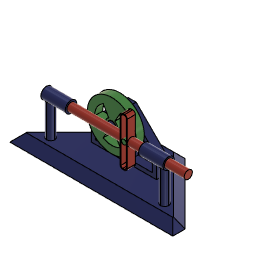
scotch yoke (Autodesk Fusion 360 design; units mm, degrees)
Autodesk Fusion 360 part; units mm, degrees
note: some values were not read from the file. Chosen so that the rebuilt part matches the saved one: which bodies a step acts on; which face or edge a step refers to; which pieces of a blend or face edit are solid. Set by a fixed rule: which sketch regions a step uses.
sketch "Base" plane through (0, 0, 0) normal (0, 0, 1) x (1, 0, 0) in component "Base"
  line L0 (10, -5) -> (-10, -5)
  line L1 (-10, -5) -> (-10, 5)
  line L2 (-10, 5) -> (10, 5)
  line L3 (10, 5) -> (10, -5)
  line L4 (10, -5) -> (-10, 5) construction
  line L5 (-10, -5) -> (10, 5) construction
  dimension "d9" = 20
  dimension "d10" = 10
  constraint horizontal L0
  constraint perpendicular L0 L1
  constraint parallel L0 L2
  constraint parallel L1 L3
  constraint coincident L4 origin
  constraint coincident L5 origin
  measures "d9" distance of L1.end L2.end
  measures "d10" distance of L0.end L1.end
extrude "Extrude1" add sketch "Base" along normal blind 1 makes body 1 in component "Base"
sketch "Crank holder" plane through (0, 0, 1) normal (0, 0, 1) x (-1, 0, 0) in component "Base"
  line L0 (-10, -5) -> (10, -5)
  line L1 (10, -5) -> (10, 5)
  line L2 (10, 5) -> (-10, 5)
  line L3 (-10, 5) -> (-10, -5)
  line L4 (0, 0) -> (4, 0)
  line L5 (4, 0) -> (4, -1)
  line L6 (4, -1) -> (0, -1)
  line L7 (0, -1) -> (0, 0)
  line L8 (-4, -1) -> (0, -1)
  line L9 (-4, 0) -> (-4, -1)
  line L10 (0, 0) -> (-4, 0)
  line L11 (-4, 0) -> (-4, 1.5) construction
  line L12 (-4, 1.5) -> (-4, 2.5) construction
  line L13 (-4, 2.5) -> (-7.5, 2.5) construction
  line L14 (-7.5, 2.5) -> (-7.5, 1.5) construction
  line L15 (-7.5, 1.5) -> (-4, 1.5) construction
  line L16 (4, 0) -> (4, 1.5) construction
  line L17 (4, 1.5) -> (4, 2.5) construction
  line L18 (4, 2.5) -> (7.5, 2.5) construction
  line L19 (7.5, 1.5) -> (4, 1.5) construction
  line L20 (7.5, 2.5) -> (7.5, 1.5) construction
  line L21 (-7.5, 1.5) -> (-6.5, 1.5)
  line L22 (-6.5, 1.5) -> (-6.5, 2.5)
  line L23 (-6.5, 2.5) -> (-7.5, 2.5)
  line L24 (-7.5, 2.5) -> (-7.5, 1.5)
  line L25 (7.5, 1.5) -> (6.5, 1.5)
  line L26 (6.5, 1.5) -> (6.5, 2.5)
  line L27 (6.5, 2.5) -> (7.5, 2.5)
  line L28 (7.5, 2.5) -> (7.5, 1.5)
  dimension "d15" = 4
  dimension "d16" = 1
  constraint horizontal L4
  constraint vertical L5
  constraint horizontal L6
  constraint vertical L7
  constraint coincident L4.start L7.end
  constraint symmetric L4.start L7 L10.start
  constraint symmetric L4.end L7 L9.start
  constraint symmetric L5.end L7 L8.start
  constraint symmetric L6.end L7 L8.end
  constraint perpendicular L10 L11
  constraint perpendicular L10 L12
  constraint perpendicular L12 L13
  constraint perpendicular L13 L14
  constraint perpendicular L12 L15
  constraint symmetric L7 L9.start L4.end
  constraint symmetric L7 L11.end L16.end
  constraint symmetric L7 L12.end L17.end
  constraint symmetric L7 L13.end L18.end
  constraint symmetric L7 L14.end L19.start
  constraint horizontal L21
  constraint vertical L22
  constraint horizontal L23
  constraint vertical L24
  constraint coincident L13 L22.end
  constraint horizontal L25
  constraint vertical L26
  constraint horizontal L27
  constraint vertical L28
  constraint coincident L18 L26.end
  measures "d15" distance of L4.start L4.end
  measures "d16" distance of L4.start L6.end
extrude "Extrude2" add sketch "Crank holder" along normal blind 6 contours L4 L5 L6 L7 | L7 L8 L9 L10 bodies 1 in component "Base"
chamfer "Chamfer1" distance 3.5 angle 45 2 edges at (4, 0.5, 7) (-4, 0.5, 7) on bodies 1 in component "Base"
sketch "Crank pin" plane through (0, 0, 0) normal (0, -1, 0) x (1, 0, 0) in component "Base"
  line L0 (-0.5, 7) -> (-4, 3.5)
  line L1 (-4, 3.5) -> (-4, 1)
  line L2 (-4, 1) -> (4, 1)
  line L3 (4, 1) -> (4, 3.5)
  line L4 (4, 3.5) -> (0.5, 7)
  line L5 (0.5, 7) -> (-0.5, 7)
  circle A0 centre (0, 5.5) radius 0.5
  line L6 (0, 5.5) -> (0, 1) construction
  dimension "d20" = 1
  constraint coincident A0.centre L6.start
  constraint midpoint L2 L6.end
  constraint perpendicular L2 L6
  measures "d20" diameter of A0
extrude "Extrude3" add sketch "Crank pin" along normal blind 1.5 contours A0 bodies 1 in component "Base"
extrude "Extrude4" add sketch "Crank holder" along normal blind 4.5 contours L21 L22 L23 L24 | L25 L26 L27 L28 bodies 1 in component "Base"
sketch "Crank" plane through (0, 0, 0) normal (0, -1, 0) x (1, 0, 0) in component "Crank"
  circle A0 centre (0, 5.5) radius 0.5
  line L0 (-0.5, 7) -> (-4, 3.5)
  line L1 (-4, 3.5) -> (-4, 1)
  line L2 (-4, 1) -> (4, 1)
  line L3 (4, 1) -> (4, 3.5)
  line L4 (4, 3.5) -> (0.5, 7)
  line L5 (0.5, 7) -> (-0.5, 7)
  circle A1 centre (0, 5.5) radius 3
  dimension "d25" = 6
  constraint concentric A0 A1
  measures "d25" diameter of A1
extrude "Extrude1'" add sketch "Crank" along normal blind 1.5 and the other way blind -0.5 separate body contours L0 L4 L5 A1 | L0 L4 L5 A1 makes body 2 in component "Crank"
sketch "holder" plane through (0, -0.5, 0) normal (0, 1, 0) x (-1, 0, 0) in component "Crank"
  circle A0 centre (0, 5.5) radius 0.5
  circle A1 centre (0, 5.5) radius 3
  circle A2 centre (0, 5.5) radius 0.5996
  dimension "d30" = 0.0996
extrude "Extrude2'" add sketch "holder" along normal blind 0.5 contours A2 bodies 2 in component "Crank"
move_face "OffsetFaces1" offset -0.02 1 faces at (0.4975, -1.1667, 5.4502) on bodies 2 in component "Crank"
sketch "pin" plane through (0, -1.5, 0) normal (0, -1, 0) x (1, 0, 0) in component "Crank"
  circle A0 centre (0, 5.5) radius 0.52
  circle A1 centre (0, 5.5) radius 3
  line L0 (0, 5.5) -> (3, 5.5) construction
  circle A2 centre (2.4981, 5.5) radius 0.25
  dimension "d34" = 0.5
  constraint coincident A0.centre A1.centre
  constraint coincident A1 L0.end
  constraint horizontal L0
  constraint coincident L0 A2.centre
  measures "d34" diameter of A2
extrude "Extrude3'" add sketch "pin" along normal blind 1 contours A2 bodies 2 in component "Crank"
sketch "slider" plane through (0, -1.5, 0) normal (0, -1, 0) x (1, 0, 0) in component "Slider"
  circle A0 centre (2.4981, 5.5) radius 0.25
  circle A1 centre (0, 5.5) radius 0.52
  circle A2 centre (0, 5.5) radius 3
  line L0 (2.6081, 8.36) -> (2.3881, 8.36)
  line L1 (2.1681, 8.14) -> (2.1681, 2.86)
  line L2 (2.3881, 2.64) -> (2.6081, 2.64)
  line L3 (2.8281, 2.86) -> (2.8281, 8.14)
  line L4 (2.8281, 8.36) -> (2.1681, 2.64) construction
  line L5 (2.1681, 8.36) -> (2.8281, 2.64) construction
  arc A3 (2.3881, 8.36) -> (2.1681, 8.14) centre (2.3881, 8.14) ccw
  arc A4 (2.8281, 8.14) -> (2.6081, 8.36) centre (2.6081, 8.14) ccw
  arc A5 (2.6081, 2.64) -> (2.8281, 2.86) centre (2.6081, 2.86) ccw
  arc A6 (2.1681, 2.86) -> (2.3881, 2.64) centre (2.3881, 2.86) ccw
  line L6 (2.3881, 2.53) -> (2.6081, 2.53)
  arc A7 (2.6081, 2.53) -> (2.9381, 2.86) centre (2.6081, 2.86) ccw
  line L7 (2.9381, 2.86) -> (2.9381, 8.14)
  arc A8 (2.9381, 8.14) -> (2.6081, 8.47) centre (2.6081, 8.14) ccw
  line L8 (2.6081, 8.47) -> (2.3881, 8.47)
  arc A9 (2.3881, 8.47) -> (2.0581, 8.14) centre (2.3881, 8.14) ccw
  line L9 (2.0581, 8.14) -> (2.0581, 2.86)
  arc A10 (2.0581, 2.86) -> (2.3881, 2.53) centre (2.3881, 2.86) ccw
  point P0 (2.4981, 5.5)
  constraint horizontal L0
  constraint perpendicular L0 L1
  constraint parallel L0 L2
  constraint parallel L1 L3
  constraint coincident L4 P0
  constraint coincident L5 P0
  constraint coincident P0 A0.centre
  constraint coincident L5.start L1
  constraint coincident L5.start L0
  constraint tangent L1 A3
  constraint tangent L0 A3
  constraint coincident L4.start L0
  constraint coincident L4.start L3
  constraint tangent L0 A4
  constraint tangent L3 A4
  constraint equal A3 A4
  constraint coincident L5.end L3
  constraint coincident L5.end L2
  constraint tangent L3 A5
  constraint tangent L2 A5
  constraint equal A3 A5
  constraint coincident L4.end L1
  constraint coincident L4.end L2
  constraint tangent L1 A6
  constraint tangent L2 A6
  constraint equal A3 A6
  constraint parallel L2 L6
  constraint concentric A5 A7
  constraint parallel L3 L7
  constraint concentric A4 A8
  constraint parallel L0 L8
  constraint concentric A3 A9
  constraint parallel L1 L9
  constraint concentric A6 A10
  constraint tangent L6 A10
  constraint tangent L6 A7
  constraint tangent A7 L7
  constraint tangent L9 A10
  constraint tangent L7 A8
  constraint tangent A8 L8
  constraint tangent L8 A9
  constraint tangent A9 L9
extrude "Extrude1''" add sketch "slider" along normal blind 1 and the other way blind 0 separate body contours A2 L3 L7 | A2 L0 L1 L3 A3 A4 L7 A8 L8 A9 L9 | A2 L1 L2 L3 A5 A6 L6 A7 L7 L9 A10 | A2 L1 L9 makes body 3 in component "Slider"
sketch "pistons" plane through (2.9381, 0, 0) normal (1, 0, 0) x (0, 1, 0) in component "Slider"
  line L0 (-1.5, 2.86) -> (-1.5, 8.14)
  line L1 (-1.5, 8.14) -> (-2.5, 8.14)
  line L2 (-2.5, 8.14) -> (-2.5, 2.86)
  line L3 (-2.5, 2.86) -> (-1.5, 2.86)
  line L4 (-2, 8.14) -> (-2, 2.86) construction
  circle A0 centre (-2, 5.5) radius 0.5
  dimension "d49" = 1
  constraint midpoint L1 L4.start
  constraint midpoint L3 L4.end
  constraint midpoint L4 A0.centre
  measures "d49" diameter of A0
extrude "Extrude2''" add sketch "pistons" along normal blind 5 contours A0 bodies 3 in component "Slider"
extrude "Extrude3''" add sketch "pistons" along normal blind -0.7 and the other way blind 5.7 contours A0 bodies 3 in component "Slider"
sketch "piston holder" plane through (7.5, 0, 0) normal (1, 0, 0) x (0, 1, 0) in component "Base"
  line L0 (-2.5, 1) -> (-1.5, 1)
  line L1 (-1.5, 1) -> (-1.5, 5.5)
  line L2 (-1.5, 5.5) -> (-2.5, 5.5)
  line L3 (-2.5, 5.5) -> (-2.5, 1)
  circle A0 centre (-2, 5.5) radius 0.5
  circle A1 centre (-2, 5.5) radius 0.7
  dimension "d56" = 1
  dimension "d57" = 0.2
  constraint midpoint L2 A0.centre
  measures "d56" diameter of A0
extrude "Extrude5" cut sketch "piston holder" against normal blind 1 contours L2 A0 | L2 A0 bodies 1 in component "Base"
extrude "Extrude6" add sketch "piston holder" along normal blind 0 and the other way blind 1 contours L1 L3 A0 A1 | L1 L3 A0 A1 bodies 1 in component "Base"
move_face "OffsetFaces1'" offset -0.03 1 faces at (6.8333, -2.4975, 5.5498) on bodies 1 in component "Base"
extrude "Extrude7" cut sketch "piston holder" against normal blind 15 contours L2 A0 | L2 A0 bodies 1 in component "Base"
extrude "Extrude8" add sketch "piston holder" along normal blind -15 and the other way blind 14 contours L1 L3 A0 A1 | L1 L3 A0 A1 bodies 1 in component "Base"
extrude "Extrude4'" cut 1 faces at (2.2381, -1.8165, 5.3449) along direction (-1, 0, 0) blind 0.07 on bodies 3 bodies 3 in component "Slider"
extrude "Extrude5'" add 1 faces at (-2.7619, -2.1035, 5.7933) along direction (-1, 0, 0) blind 0.07 on bodies 3 bodies 3 in component "Slider"
sketch "extend holder left" plane through (-6.5, 0, 0) normal (1, 0, 0) x (0, 1, 0) in component "Base"
  circle A0 centre (-2, 5.5) radius 0.5
  arc A1 (-1.5, 5.0101) -> (-2.5, 5.0101) centre (-2, 5.5) ccw
  line L0 (-2.5, 5.0101) -> (-2.5, 1)
  line L1 (-2.5, 1) -> (-1.5, 1)
  line L2 (-1.5, 1) -> (-1.5, 5.0101)
  circle A2 centre (-2, 5.5) radius 0.5
  circle A3 centre (-2, 5.5) radius 0.7
  constraint concentric A0 A2
  constraint concentric A2 A3
extrude "Extrude9" add sketch "extend holder left" along normal blind 2 contours A1 A3 bodies 1 in component "Base"
sketch "extend holder right" plane through (6.5, 0, 0) normal (-1, 0, 0) x (0, -1, 0) in component "Base"
  circle A0 centre (2, 5.5) radius 0.53
  arc A1 (2.5, 5.0101) -> (1.5, 5.0101) centre (2, 5.5) ccw
  line L0 (1.5, 5.0101) -> (1.5, 1)
  line L1 (1.5, 1) -> (2.5, 1)
  line L2 (2.5, 1) -> (2.5, 5.0101)
  circle A2 centre (2, 5.5) radius 0.53
  circle A3 centre (2, 5.5) radius 0.7
  constraint concentric A0 A2
  constraint concentric A2 A3
extrude "Extrude10" add sketch "extend holder right" along normal blind 2 contours A1 A3 bodies 1 in component "Base"
extrude "Extrude6'" add 1 faces at (7.9381, -1.8165, 5.3449) along direction (1, 0, 0) blind 2 on bodies 3 bodies 3 in component "Slider"
extrude "Extrude7'" add 1 faces at (-2.8319, -2.1035, 5.7933) along direction (-1, 0, 0) blind 2 on bodies 3 bodies 3 in component "Slider"
move_face "OffsetFaces2" offset 0.05 1 faces at (2.7478, -2.1667, 5.4875) on bodies 2 in component "Crank"
sketch "remove extra material" plane through (0, -1.5, 0) normal (0, -1, 0) x (1, 0, 0) in component "Crank"
  circle A0 centre (2.4981, 5.5) radius 0.3
  circle A1 centre (0, 5.5) radius 0.52
  circle A2 centre (0, 5.5) radius 3
  circle A3 centre (0, 5.5) radius 2.1
  line L0 (0, 5.5) -> (0, 7.6) construction
  line L1 (0.375, 6.1495) -> (1.05, 7.3187)
  line L2 (-0.75, 5.5) -> (-2.1, 5.5)
  line L3 (0.75, 5.5) -> (2.1, 5.5)
  line L4 (0.375, 4.8505) -> (1.05, 3.6813)
  circle A4 centre (0, 5.5) radius 0.75
  line L5 (-0.375, 6.1495) -> (-1.05, 7.3187)
  line L6 (-0.375, 4.8505) -> (-1.05, 3.6813)
  dimension "d89" = 30
  dimension "d92" = 1.5
  constraint concentric A1 A3
  constraint coincident A1.centre A2.centre
  constraint coincident A3 L0.end
  constraint vertical L0
  constraint coincident A3 L1.end
  constraint coincident A3 L5.end
  constraint concentric A3 A4
  constraint coincident A4 L5.start
  constraint coincident A4 L2.start
  constraint coincident A4 L6.start
  constraint coincident A4 L1.start
  constraint coincident A4 L4.start
  constraint coincident A4 L3.start
  measures "d89" angle of L0 L1
  measures "d92" diameter of A4
extrude "Extrude4''" cut sketch "remove extra material" against normal blind 1 contours A3 L1 L3 A4 | A3 L4 A4 L6 | A3 L2 A4 L5 bodies 2 in component "Crank"
fillet "Fillet1" radius 0.49 4 edges at (-7.5, -2.5, 3.0051) (-7.5, -1.5, 3.0051) (-6.5, -2.5, 3.0051) (-6.5, -1.5, 3.0051) on bodies 1 in component "Base"
fillet "Fillet2" radius 0.49 4 edges at (6.5, -1.5, 3.0051) (6.5, -2.5, 3.0051) (7.5, -2.5, 3.0051) (7.5, -1.5, 3.0051) on bodies 1 in component "Base"
sketch "remove extra material (2)" plane through (0, 1, 0) normal (0, 1, 0) x (-1, 0, 0) in component "Base"
  line L0 (4, 3.5) -> (0.5, 7)
  line L1 (0.5, 7) -> (-0.5, 7)
  line L2 (-0.5, 7) -> (-4, 3.5)
  line L3 (-4, 3.5) -> (-4, 1)
  line L4 (-4, 1) -> (4, 1)
  line L5 (4, 1) -> (4, 3.5)
  line L6 (-3.5, 1.5) -> (3.5, 1.5)
  line L7 (3.5, 1.5) -> (3.5, 3.2929)
  line L8 (3.5, 3.2929) -> (0.2929, 6.5)
  line L9 (0.2929, 6.5) -> (-0.2929, 6.5)
  line L10 (-0.2929, 6.5) -> (-3.5, 3.2929)
  line L11 (-3.5, 3.2929) -> (-3.5, 1.5)
  circle A0 centre (0, 5.5) radius 0.75
  line L12 (-0.75, 6.0429) -> (-0.75, 1.5)
  line L13 (0.75, 6.0429) -> (0.75, 1.5)
  dimension "d99" = -0.5
  dimension "d100" = 1.5
  constraint coincident L10 L12.start
  constraint coincident L6 L12.end
  constraint perpendicular L6 L12
  constraint coincident L8 L13.start
  constraint coincident L6 L13.end
  constraint perpendicular L6 L13
  constraint tangent A0 L12
  constraint tangent A0 L13
  measures "d100" diameter of A0
extrude "Extrude11" cut sketch "remove extra material (2)" against normal blind 1 contours L6 L10 L11 L12 | L6 L7 L8 L13 bodies 1 in component "Base"
split "Split1" by plane through (0, 0, 1) normal (0, 0, 1) bodies 1 makes body 4 at (-5.8333, -2.4994, 5.4751) makes body 5 at (-0.25, 1, 4.5286) makes body 6 at (6.1667, -1.4471, 5.0707) in component "Base"
combine "Combine1" operation add target body 1 tool bodies 5 in component "Base"
extrude "Extrude12" cut 2 faces at (-7.1667, -1.9967, 1) (6.8333, -1.9967, 1) along direction (0, 0, -1) blind 0.8 on bodies 4 6 bodies 1 in component "Base"
extrude "Extrude13" add 2 faces at (6.8333, -1.9967, 1) (-7.1667, -1.9967, 1) along direction (0, 0, -1) blind 0.8 on bodies 4 6 bodies 6 4 in component "Base"
copy_body "CutPasteBodies1" bodies 4 removing the originals makes body 7 in component "Piston Holders"
copy_body "CutPasteBodies2" bodies 6 removing the originals makes body 8 in component "Piston Holders"
chamfer "Chamfer2" distance 7.5 angle 45 2 edges at (10, 5, 0.5) (-10, 5, 0.5) on bodies 1 in component "Base"
move_face "OffsetFaces2'" offset -1 1 faces at (3.3333, -5, 0.3333) on bodies 1 in component "Base"
chamfer "Chamfer3" distance 1 angle 45 6 edges at (6.25, 1.25, 1) (0, 5, 1) (-6.25, 1.25, 1) (-10, -3.25, 1) (0, -4, 1) (10, -3.25, 1) on bodies 1 in component "Base"
component "Base" placed x (1, 0, 0) y (0, 1, 0) z (0, 0, 1) at (0, 0, 0)
component "Crank" placed x (0.929776, 0, -0.368125) y (0, 1, 0) z (0.368125, 0, 0.929776) at (-2.0247, 0, 0.3862)
component "Slider" placed x (1, 0, 0) y (0, 1, 0) z (0, 0, 1) at (-0.1454, 0, 0)
component "Piston Holders" placed x (1, 0, 0) y (0, 1, 0) z (0, 0, 1) at (0, 0, 0)
named bodies: "base", "crank", "base (1)", "base (2)", "base (3)", "left", "right"
